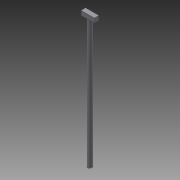
# Autodesk Inventor part: EE_Arm-Rod-Rev1
Saved by Autodesk Inventor 2015 (Build 190159000, 159)
## iProperties
Created: 2016-12-22
Part Number: EE_Arm-Rod-Rev1
Material: Generic
Document SubType Name: Modeling
Designer: Guy
Density: 1 g/cm^3
Appearance: Default
Author: Guy
Autodesk Inventor part; units mm, degrees
ref_plane "YZ Plane" through (0, 0, 0) normal (1, 0, 0) x (0, 1, 0)
ref_plane "XZ Plane" through (0, 0, 0) normal (0, 1, 0) x (-1, 0, 0)
ref_plane "XY Plane" through (0, 0, 0) normal (0, 0, 1) x (1, 0, 0)
sketch "Sketch1" plane through (0, 0, 0) normal (0, 0, 1) x (1, 0, 0)
  circle A0 centre (0, 0) radius 5
  dimension "d0" = 10
  constraints: 1 centre point, 1 coincident
  measures "d0" diameter of A0
extrude "Extrusion1" add sketch "Sketch1" along normal blind 300
sketch "Sketch2" plane through (0, 0, 0) normal (1, 0, 0) x (0, 1, 0)
  line L0 (-5, 0) -> (-5, 300) projected
  line L1 (5, 0) -> (5, 300) projected
  line L2 (5, 300) -> (-5, 300) projected
  line L3 (-5, 300) -> (5, 300)
  line L4 (5, 300) -> (5, 290)
  line L5 (5, 290) -> (-5, 290)
  line L6 (-5, 290) -> (-5, 300)
  point P0 (0, 0)
  dimension "d3" = 10
  constraints: 8 end point, 2 parallel, 1 horizontal, 1 perpendicular, 1 point on line
  measures "d3" distance between parallel lines of L5 L2
extrude "Extrusion2" add sketch "Sketch2" along normal mid plane 30
ref_plane "Work Plane1" through (-15, 0, 300) normal (0, -1, 0) x (1, 0, 0)
sketch "Sketch3" plane through (-15, 0, 300) normal (0, -1, 0) x (1, 0, 0)
  line L0 (0, 0) -> (30, 0) projected
  line L1 (30, -10) -> (30, 0) projected
  line L2 (15, -10) -> (30, -10) projected
  line L3 (0, -10) -> (15, -10) projected
  line L4 (0, 0) -> (0, -10) projected
  line L5 (15, -10) -> (15, -10) projected
  line L6 (15, -10) -> (15, -10) projected
  line L7 (10, -300) -> (20, -300) projected
  line L8 (20, -300) -> (20, -10) projected
  line L9 (10, -300) -> (20, -298.2367)
  line L10 (10, -300) -> (20, -300) projected
  line L11 (20, -298.2367) -> (20, -300)
  line L12 (10, -300) -> (20, -300)
  line L13 (10, -300) -> (10, -10) projected
  point P0 (15, -300)
  dimension "d10" = 10
  constraints: 6 end point, 2 collinear, 1 point on line
  measures "d10" angle of L9 L7
extrude "Extrusion3" cut sketch "Sketch3" along normal through all both and the other way through all contours L9 L8 L7
body "Solid1"
